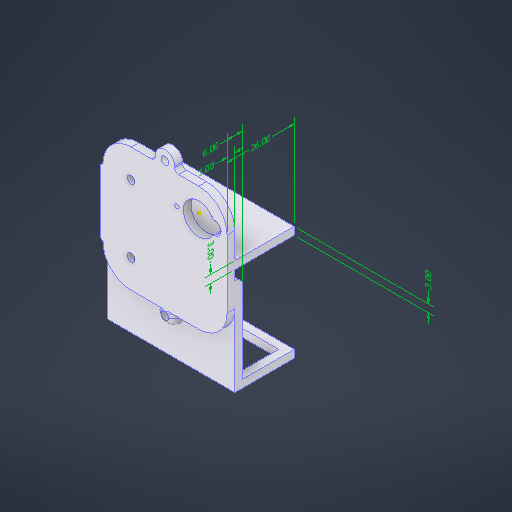
# Autodesk Inventor part: sheet4
Saved by Autodesk Inventor 2025.3 (Build 293356000, 356)
## iProperties
Created: 2016-01-21
Part Number: sheet4
Material: ABS Plastic
Document SubType Name: Modeling
Designer: Nanjar
Density: 1.06 g/cm^3
Appearance: Cool White
Author: Nanjar
Autodesk Inventor part; units mm, degrees
ref_plane "YZ Plane" through (0, 0, 0) normal (1, 0, 0) x (0, 1, 0)
ref_plane "XZ Plane" through (0, 0, 0) normal (0, 1, 0) x (-1, 0, 0)
ref_plane "XY Plane" through (0, 0, 0) normal (0, 0, 1) x (1, 0, 0)
sketch "Sketch1" plane through (0, 0, 0) normal (0, 0, 1) x (1, 0, 0)
  arc A0 (-26.3575, 9.02) -> (-37.2975, -1.92) centre (-26.3575, -1.92) ccw
  line L0 (-37.2975, -1.92) -> (-38.3625, -2.985)
  arc A1 (10.8425, -1.92) -> (-0.0975, 9.02) centre (-0.0975, -1.92) ccw
  circle A2 centre (-13.2275, 11.07) radius 1.5
  arc A3 (-9.4775, 11.07) -> (-16.9775, 11.07) centre (-13.2275, 11.07) ccw
  line L1 (-16.9775, 11.07) -> (-16.9775, 9.02)
  line L2 (-9.4775, 11.07) -> (-9.4775, 9.02)
  line L3 (-26.3575, 9.02) -> (-16.9775, 9.02)
  line L4 (-9.4775, 9.02) -> (-0.0975, 9.02)
  line L5 (10.8425, -1.92) -> (10.8425, -15)
  line L6 (-38.3625, -15) -> (10.8425, -15)
  circle A4 centre (-26.3575, -1.92) radius 1.5
  arc A5 (5.4151, 0.5728) -> (5.4151, -4.4128) centre (-0.0975, -1.92) ccw
  arc A6 (6.337, -4.4408) -> (6.337, 0.6008) centre (5.9521, -1.92) ccw
  arc A7 (5.4151, -4.4128) -> (5.4151, 0.5728) centre (5.9521, -1.92) ccw
  line L7 (-38.3625, -2.985) -> (-38.3625, -15)
  arc A8 (-37.2975, -28.08) -> (-26.3575, -39.02) centre (-26.3575, -28.08) ccw
  line L8 (-37.2975, -28.08) -> (-38.3625, -27.015)
  arc A9 (-0.0975, -39.02) -> (10.8425, -28.08) centre (-0.0975, -28.08) ccw
  circle A10 centre (-13.2275, -41.07) radius 1.5
  arc A11 (-16.9775, -41.07) -> (-9.4775, -41.07) centre (-13.2275, -41.07) ccw
  line L9 (-16.9775, -41.07) -> (-16.9775, -39.02)
  line L10 (-9.4775, -41.07) -> (-9.4775, -39.02)
  line L11 (-26.3575, -39.02) -> (-16.9775, -39.02)
  line L12 (-9.4775, -39.02) -> (-0.0975, -39.02)
  line L13 (10.8425, -28.08) -> (10.8425, -15)
  circle A12 centre (-26.3575, -28.08) radius 1.5
  arc A13 (5.4151, -25.5872) -> (5.4151, -30.5728) centre (-0.0975, -28.08) ccw
  arc A14 (6.337, -30.6008) -> (6.337, -25.5592) centre (5.9521, -28.08) ccw
  arc A15 (5.4151, -30.5728) -> (5.4151, -25.5872) centre (5.9521, -28.08) ccw
  line L14 (-38.3625, -27.015) -> (-38.3625, -15)
  dimension "d0" = 3
  dimension "d1" = 7.5
  constraints: 30 end point, 24 point on circle, 23 symmetric about line, 16 centre point, 12 coincident, 3 vertical, 2 perpendicular, 2 tangent, 8 other
  measures "d0" diameter of A2
  measures "d1" diameter of A3
extrude "Extrusion1" add sketch "Sketch1" along normal blind 3 contours L3 L1 A3 L2 L4 A1 L5 L6 L7 L0 A0 | L6 L13 A9 L12 L10 A11 L9 L11 A8 L8 L14 | A15 A14 A13
fillet "Fillet1" radius 1.5 2 edges at (-9.4775, 9.02, 1.5) (-16.9775, 9.02, 1.5)
fillet "Fillet2" radius 1.5 2 edges at (5.4151, 0.5728, 1.5) (5.4151, -4.4128, 1.5)
sketch "Sketch2" plane through (0, 0, 0) normal (0, 0, -1) x (-1, 0, 0)
  line L0 (-7.8651, -12) -> (38.3625, -12)
  line L1 (38.3625, -12) -> (38.3625, -15)
  line L2 (38.3625, -12) -> (-10.8425, -12)
  line L3 (-10.8425, -12) -> (-10.8425, -15)
  line L4 (38.3625, -15) -> (-10.8425, -15)
  constraints: 10 end point, 2 horizontal, 1 perpendicular
extrude "Extrusion2" add sketch "Sketch2" along normal blind 23
sketch "Sketch3" plane through (-38.3625, -15, 3) normal (0, -1, 0) x (1, 0, 0)
  circle A0 centre (2, -15.71) radius 0.85
  circle A1 centre (2, -15.71) radius 0.85
  circle A2 centre (30, -15.71) radius 0.85
  circle A3 centre (30, -15.71) radius 0.85
  line L0 (4.5, -21.71) -> (27.5, -21.71)
  line L1 (27.5, -21.71) -> (27.5, -9.71)
  line L2 (27.5, -21.71) -> (27.5, -9.71)
  line L3 (4.5, -9.71) -> (4.5, -21.71)
  line L4 (27.5, -9.71) -> (4.5, -9.71)
  line L5 (4.5, -9.71) -> (4.5, -21.71)
  line L6 (4.5, -21.71) -> (27.5, -21.71)
  line L7 (0, -26) -> (0, 0) projected
  line L8 (49.205, -26) -> (0, -26) projected
  constraints: 14 end point, 4 centre point, 2 coincident, 2 collinear, 1 perpendicular, 1 vertical
extrude "Extrusion3" [suppressed]
sketch "Sketch4" plane through (-38.3625, -15, 3) normal (0, -1, 0) x (1, 0, 0)
  line L0 (32, -26) -> (32, -9.71)
  line L1 (32, -9.71) -> (49.205, -9.71)
  line L2 (49.205, -26) -> (49.205, -9.71)
  line L3 (49.205, -26) -> (32, -26)
  constraints: 8 end point, 1 perpendicular
extrude "Extrusion4" [suppressed]
fillet "Fillet3" radius 0.8 1 edges at (-13.76, -12, 0)
sketch "Sketch5" plane through (0, 0, 0) normal (0, 0, -1) x (-1, 0, 0)
  circle A0 centre (8.5925, -1.92) radius 0.85
  line L0 (-10.8425, -15) -> (38.3625, -15) projected
  line L1 (38.3625, -2.985) -> (38.3625, -11.2) projected
  point P0 (0, 0)
  point P1 (6.3625, -15)
  dimension "d20" = 1.7
  dimension "d21" = 13.08
  dimension "d22" = 29.77
  constraints: 1 centre point
  measures "d20" diameter of A0
  measures "d21" distance from line of L0 A0.centre
  measures "d22" distance from line of L1 A0.centre
extrude "Extrusion5" cut sketch "Sketch5" against normal through all
sketch "Sketch6" plane through (-38.3625, -15, 2.2) normal (0, -1, 0) x (1, 0, 0)
  line L0 (39.65, -19.16) -> (36.65, -19.16)
  line L1 (36.65, -19.16) -> (36.65, -8.66)
  line L2 (36.65, -8.66) -> (39.65, -8.66)
  line L3 (39.65, -8.66) -> (39.65, -19.16)
  line L4 (39.65, -19.16) -> (36.65, -8.66) construction
  line L5 (36.65, -19.16) -> (39.65, -8.66) construction
  line L6 (49.205, -25.2) -> (0, -25.2) projected
  line L7 (49.205, -25.2) -> (49.205, 0) projected
  point P0 (38.3625, -2.2)
  point P1 (38.15, -13.91)
  dimension "d28" = 3
  dimension "d29" = 10.5
  dimension "d30" = 6.04
  dimension "d31" = 9.555
  constraints: 12 end point, 2 midpoint, 2 parallel, 1 horizontal, 1 perpendicular
  measures "d28" distance of L1.end L2.end
  measures "d29" distance of L0.end L1.end
  measures "d30" distance between parallel lines of L6 L0
  measures "d31" distance between parallel lines of L7 L3
extrude "Extrusion6" [suppressed]
sketch "Sketch7" plane through (-38.3625, -15, 2.2) normal (0, -1, 0) x (1, 0, 0)
  line L0 (49.205, -3) -> (49.205, -25.2) projected
  line L1 (49.205, -25.2) -> (44.205, -25.2)
  line L2 (44.205, -25.2) -> (44.205, -4.7305)
  line L3 (44.205, -4.7305) -> (49.205, -4.7305)
  line L4 (49.205, -4.7305) -> (49.205, -25.2)
  line L5 (39.65, -8.66) -> (39.65, -19.16) projected
  point P0 (38.3625, -2.2)
  dimension "d34" = 4.555
  constraints: 8 end point, 2 parallel, 1 horizontal, 1 perpendicular
  measures "d34" distance between parallel lines of L5 L2
extrude "Extrusion7" [suppressed]
sketch "Sketch10" plane through (0, 0, 3) normal (0, 0, 1) x (1, 0, 0)
  point P0 (0, 0)
sketch "Sketch11" plane through (0, 0, 0) normal (0, 0, -1) x (-1, 0, 0)
  circle A0 centre (13.2275, -41.07) radius 1.5 projected
  circle A1 centre (13.2275, -41.07) radius 1.5
  line L0 (-10.8425, -28.08) -> (-10.8425, -1.92) projected
  line L1 (38.3625, -15) -> (38.3625, -27.015) projected
  line L2 (-10.8425, -15) -> (38.3625, -15)
  line L3 (38.3625, -15) -> (38.3625, -56.2739)
  line L4 (38.3625, -56.2739) -> (-10.8425, -56.2739)
  line L5 (-10.8425, -56.2739) -> (-10.8425, -28.3143)
  line L6 (-10.8425, -28.3143) -> (-10.8425, -15)
  line L7 (-10.8425, -18.6924) -> (38.3625, -18.6924)
  point P0 (0, 0)
  constraints: 12 end point, 4 perpendicular, 2 collinear, 2 point on line, 1 centre point, 1 coincident, 1 midpoint
extrude "Extrusion8" add sketch "Sketch11" along normal blind 3 contours L0 L7 L1 L3 L4 L5 L6
sketch "Sketch12" plane through (0, 0, -3) normal (0, 0, -1) x (-1, 0, 0)
  line L0 (-10.8425, -56.2739) -> (38.3625, -56.2739) projected
  line L1 (-10.8425, -56.2739) -> (-10.8425, -53.2739)
  line L2 (-10.8425, -28.08) -> (-10.8425, -56.2739) projected
  line L3 (-10.8425, -53.2739) -> (38.3625, -53.2739)
  line L4 (38.3625, -56.2739) -> (38.3625, -27.015) projected
  line L5 (38.3625, -53.2739) -> (38.3625, -56.2739)
  line L6 (38.3625, -56.2739) -> (-10.8425, -56.2739)
  point P0 (0, 0)
  dimension "d58" = 3
  constraints: 8 end point, 2 perpendicular, 2 point on line, 1 vertical
  measures "d58" distance of L0.start L1.end
extrude "Extrusion9" add sketch "Sketch12" along normal blind 20
sketch "Sketch13" plane through (-38.3625, -56.2739, 0) normal (0, -1, 0) x (1, 0, 0)
  line L0 (1.065, 0) -> (0, 0) projected
  line L1 (0, 0) -> (3, -3)
  line L2 (0, -3) -> (49.205, -3) projected
  line L3 (0, 0) -> (4.2426, 0) construction
  line L4 (49.205, 0) -> (49.205, -23) projected
  line L5 (49.205, -23) -> (49.205, -20)
  line L6 (49.205, -23) -> (46.205, -20)
  line L7 (49.205, -23) -> (53.4476, -23) construction
  line L8 (3, -3) -> (46.205, -3)
  line L9 (46.205, -3) -> (46.205, -20)
  line L10 (46.205, -20) -> (3, -20)
  line L11 (3, -20) -> (3, -3)
  point P0 (38.3625, 0)
  dimension "d66" = 45
  dimension "d67" = 3
  dimension "d68" = 3
  dimension "d69" = 135
  constraints: 18 end point, 3 horizontal, 2 equal length, 2 parallel, 2 point on line, 1 perpendicular
  measures "d66" angle of L1 L3
  measures "d67" horizontal distance of L0.end L1.end
  measures "d68" distance of L4.end L5.end
  measures "d69" angle of L7 L6
extrude "Extrusion10" cut sketch "Sketch13" against normal blind 20 contours L2 L9 L10 L11
sketch "Sketch14" plane through (-35.3625, -56.2739, -20) normal (0, 0, 1) x (1, 0, 0)
  line L0 (43.205, 0) -> (0, 0) projected
  line L1 (43.205, 0) -> (0, 0)
  line L2 (0, 0) -> (21.6, 0)
  line L3 (21.6, 0) -> (18.6, 0)
  line L4 (18.6, 0) -> (18.6, 3)
  line L5 (0, 3) -> (43.205, 3) projected
  line L6 (18.6, 3) -> (24.6, 3)
  line L7 (24.6, 3) -> (24.6, 0)
  line L8 (21.6, 0) -> (24.6, 0)
  point P0 (35.3625, 56.2739)
  point P1 (24.6, 0)
  point P2 (24.6, 3)
  point P3 (18.6, 0)
  dimension "d72" = 21.6
  dimension "d73" = 3
  dimension "d74" = 6
  constraints: 14 end point, 4 point on line, 3 perpendicular, 2 collinear
  measures "d72" distance of L0.end L2.end
  measures "d73" distance of L2.end L3.end
  measures "d74" distance of L4.end L6.end
extrude "Extrusion11" add sketch "Sketch14" along normal blind 20
fillet "Fillet4" radius 3 3 edges at (-9.4775, -40.045, 3) (-16.9775, -40.045, 3) (-13.2275, -44.82, 3)
sketch "Sketch15" plane through (-38.3625, -56.2739, 0) normal (0, -1, 0) x (1, 0, 0)
  line L0 (21.6, -20) -> (21.6, -3) projected
  line L1 (27.6, -20) -> (46.205, -20) projected
  line L2 (21.6, -20) -> (27.6, -20)
  line L3 (27.6, -3) -> (21.6, -3) projected
  circle A0 centre (24.6, -11.5) radius 1.5
  point P0 (38.3625, 0)
  dimension "d78" = 3
  constraints: 2 end point, 1 centre point, 1 collinear
  measures "d78" diameter of A0
extrude "Extrusion12" cut sketch "Sketch15" against normal blind 20
fillet "Fillet5" radius 3 1 edges at (-13.76, -18.6924, -3)
body "Solid1"
